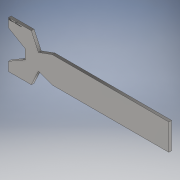
# Autodesk Inventor part: Spare Blade (In Blade Holder)
Saved by Autodesk Inventor 2021 (Build 250183000, 183)
## iProperties
Created: 2021-05-04
Part Number: Spare Blade (In Blade Holder)
Material: Generic
Document SubType Name: Modeling
Designer: AHUJA
Density: 1 g/cm^3
Appearance: Default
Author: AHUJA
Autodesk Inventor part; units mm, degrees
ref_plane "YZ Plane" through (0, 0, 0) normal (1, 0, 0) x (0, 1, 0)
ref_plane "XZ Plane" through (0, 0, 0) normal (0, 1, 0) x (-1, 0, 0)
ref_plane "XY Plane" through (0, 0, 0) normal (0, 0, 1) x (1, 0, 0)
sketch "Sketch1" plane through (0, 0, 0) normal (0, 0, 1) x (1, 0, 0)
  line L0 (0, 0) -> (80, 0)
  line L1 (80, 0) -> (80, 18)
  line L2 (80, 18) -> (0, 18)
  line L3 (0, 18) -> (0, 0)
  line L4 (0, 25) -> (-30, 25)
  line L5 (-30, -7) -> (0, -7)
  line L6 (0, -7) -> (0, 25)
  line L7 (0, 18) -> (-9.3969, 14.5798)
  line L8 (0, 18) -> (10, 18) construction
  line L9 (0, 0) -> (-9.3969, 3.4202)
  line L10 (0, 0) -> (10, 0) construction
  line L11 (-9.3969, 14.5798) -> (-14.2559, 25)
  line L12 (-9.3969, 14.5798) -> (2.1005, 14.5798) construction
  line L13 (-9.3969, 3.4202) -> (-14.2559, -7)
  line L14 (-9.3969, 3.4202) -> (2.1005, 3.4202) construction
  line L15 (-30, 25) -> (-30, 19)
  line L16 (-30, 19) -> (-18.3849, 12.294)
  line L17 (-30, -7) -> (-30, -1)
  line L18 (-30, -1) -> (-18.3849, 5.706)
  line L19 (-18.3849, 5.706) -> (-18.3849, 12.294)
  line L20 (-30, 25) -> (-30, 19)
  line L21 (-30, -1) -> (-30, -7)
  dimension "d0" = 80
  dimension "d1" = 18
  dimension "d2" = 30
  dimension "d3" = 0
  dimension "d4" = 7
  dimension "d5" = 7
  dimension "d6" = 160
  dimension "d7" = 160
  dimension "d8" = 10
  dimension "d9" = 10
  dimension "d10" = 115
  dimension "d11" = 115
  dimension "d12" = 6
  dimension "d13" = 120
  dimension "d14" = 6
  dimension "d15" = 120
  dimension "d16" = 30
  constraints: 44 end point, 6 horizontal, 6 parallel, 4 equal length, 3 perpendicular, 2 point on line
  measures "d0" distance of L1.end L2.end
  measures "d1" distance of L0.end L1.end
  measures "d2" distance of L4.start L4.end
  measures "d3" distance between parallel lines of L3 L6
  measures "d4" distance between parallel lines of L2 L4
  measures "d5" distance between parallel lines of L5 L0
  measures "d6" angle of L7 L8
  measures "d7" angle of L10 L9
  measures "d8" distance of L2.end L7.end
  measures "d9" distance of L0.start L9.end
  measures "d10" angle of L12 L11
  measures "d11" angle of L13 L14
  measures "d12" distance of L4.end L15.end
  measures "d13" angle of L16 L15
  measures "d14" distance of L5.start L17.end
  measures "d15" angle of L17 L18
  measures "d16" distance of L5.start L5.end
extrude "Extrusion1" add sketch "Sketch1" along normal blind 1.905 contours L3 L2 L1 L0 | L9 L13 L5 L17 L18 L19 L16 L15 L4 L11 L7 L3
sketch "Sketch2" plane through (0, 0, 1.905) normal (0, 0, 1) x (1, 0, 0)
  line L0 (-30.0598, 24.874) -> (-18.1328, 24.874) construction
  line L1 (-18.1328, 24.874) -> (-18.1328, 20.2492) construction
  line L2 (-18.1328, 20.2492) -> (-30.0598, 20.2492) construction
  line L3 (-30.0598, 20.2492) -> (-30.0598, 24.874) construction
  spline S0 degree 2 poles (-29.0996, 24.3152) (-28.6048, 24.816) (-28.4664, 24.816) knots 0 0 0 1 1 1
  spline S1 degree 2 poles (-28.4664, 24.816) (-28.4084, 24.816) (-28.4084, 24.7615) knots 0 0 0 1 1 1
  spline S2 degree 2 poles (-28.4084, 24.7615) (-28.4084, 24.7105) (-28.4499, 24.6482) knots 0 0 0 1 1 1
  spline S3 degree 2 poles (-28.4499, 24.6482) (-28.4811, 24.6041) (-28.8236, 24.2451) knots 0 0 0 1 1 1
  spline S4 degree 2 poles (-28.8236, 24.2451) (-29.1091, 23.9285) (-29.1091, 23.8731) knots 0 0 0 1 1 1
  spline S5 degree 2 poles (-29.1091, 23.8731) (-29.1091, 23.8541) (-29.0538, 23.8498) (-29.0538, 23.8437) knots 0 0 0 1 2 2 2
  spline S6 degree 2 poles (-29.0538, 23.8437) (-29.0538, 23.8238) (-29.097, 23.8238) knots 0 0 0 1 1 1
  spline S7 degree 2 poles (-29.097, 23.8238) (-29.1584, 23.8238) (-29.1584, 23.8818) knots 0 0 0 1 1 1
  spline S8 degree 2 poles (-29.1584, 23.8818) (-29.1584, 23.989) (-28.892, 24.2857) knots 0 0 0 1 1 1
  spline S9 degree 2 poles (-28.892, 24.2857) (-28.7986, 24.3904) (-28.5382, 24.6517) knots 0 0 0 1 1 1
  spline S10 degree 2 poles (-28.5382, 24.6517) (-28.4491, 24.7399) (-28.4491, 24.7754) knots 0 0 0 1 1 1
  spline S11 degree 2 poles (-28.4491, 24.7754) (-28.4491, 24.7892) (-28.4629, 24.7892) knots 0 0 0 1 1 1
  spline S12 degree 2 poles (-28.4629, 24.7892) (-28.5122, 24.7892) (-28.7406, 24.5998) knots 0 0 0 1 1 1
  spline S13 degree 2 poles (-28.7406, 24.5998) (-28.9231, 24.4475) (-29.0131, 24.3575) knots 0 0 0 1 1 1
  spline S14 degree 2 poles (-29.0131, 24.3575) (-29.0996, 24.271) (-29.2406, 24.1136) knots 0 0 0 1 1 1
  spline S15 degree 2 poles (-29.2406, 24.1136) (-29.4941, 23.829) (-29.5018, 23.829) knots 0 0 0 1 1 1
  spline S16 degree 2 poles (-29.5018, 23.829) (-29.5122, 23.829) (-29.5416, 23.8558) (-29.5416, 23.8671) knots 0 0 0 1 2 2 2
  spline S17 degree 2 poles (-29.5416, 23.8671) (-29.5416, 23.8947) (-28.9352, 24.611) (-28.9352, 24.6681) knots 0 0 0 1 2 2 2
  spline S18 degree 2 poles (-28.9352, 24.6681) (-28.9352, 24.6828) (-28.9491, 24.6828) knots 0 0 0 1 1 1
  spline S19 degree 2 poles (-28.9491, 24.6828) (-28.9863, 24.6828) (-29.1377, 24.5686) knots 0 0 0 1 1 1
  spline S20 degree 2 poles (-29.1377, 24.5686) (-29.2778, 24.4631) (-29.4456, 24.303) knots 0 0 0 1 1 1
  line L4 (-29.4456, 24.303) -> (-29.7345, 24.0167)
  line L5 (-29.7345, 24.0167) -> (-29.8358, 23.9077)
  spline S21 degree 2 poles (-29.8358, 23.9077) (-29.9205, 23.816) (-29.9275, 23.816) knots 0 0 0 1 1 1
  spline S22 degree 2 poles (-29.9275, 23.816) (-29.9387, 23.816) (-29.956, 23.8273) knots 0 0 0 1 1 1
  spline S23 degree 2 poles (-29.956, 23.8273) (-29.975, 23.8394) (-29.975, 23.8506) knots 0 0 0 1 1 1
  spline S24 degree 2 poles (-29.975, 23.8506) (-29.975, 23.874) (-29.796, 24.0747) knots 0 0 0 1 1 1
  line L6 (-29.796, 24.0747) -> (-29.4621, 24.4501)
  spline S25 degree 2 poles (-29.4621, 24.4501) (-29.2821, 24.6612) (-29.2821, 24.7113) knots 0 0 0 1 1 1
  spline S26 degree 2 poles (-29.2821, 24.7113) (-29.2821, 24.7295) (-29.3003, 24.7295) knots 0 0 0 1 1 1
  spline S27 degree 2 poles (-29.3003, 24.7295) (-29.3522, 24.7295) (-29.5148, 24.5972) knots 0 0 0 1 1 1
  spline S28 degree 2 poles (-29.5148, 24.5972) (-29.6368, 24.4985) (-29.8626, 24.2477) knots 0 0 0 1 1 1
  spline S29 degree 2 poles (-29.8626, 24.2477) (-29.8773, 24.2321) (-29.8859, 24.2321) knots 0 0 0 1 1 1
  spline S30 degree 2 poles (-29.8859, 24.2321) (-29.9015, 24.2321) (-29.9015, 24.2442) knots 0 0 0 1 1 1
  spline S31 degree 2 poles (-29.9015, 24.2442) (-29.9015, 24.2624) (-29.7769, 24.406) knots 0 0 0 1 1 1
  spline S32 degree 2 poles (-29.7769, 24.406) (-29.687, 24.5072) (-29.5512, 24.6205) knots 0 0 0 1 1 1
  spline S33 degree 2 poles (-29.5512, 24.6205) (-29.3747, 24.7658) (-29.296, 24.7658) knots 0 0 0 1 1 1
  spline S34 degree 2 poles (-29.296, 24.7658) (-29.2432, 24.7658) (-29.2432, 24.7079) knots 0 0 0 1 1 1
  spline S35 degree 2 poles (-29.2432, 24.7079) (-29.2432, 24.611) (-29.5001, 24.297) knots 0 0 0 1 1 1
  spline S36 degree 2 poles (-29.5001, 24.297) (-29.0615, 24.7148) (-28.9491, 24.7148) knots 0 0 0 1 1 1
  spline S37 degree 2 poles (-28.9491, 24.7148) (-28.8963, 24.7148) (-28.8963, 24.6603) knots 0 0 0 1 1 1
  spline S38 degree 2 poles (-28.8963, 24.6603) (-28.8963, 24.5747) (-29.0996, 24.3152) knots 0 0 0 1 1 1
  spline S39 degree 2 poles (-28.6091, 23.8722) (-28.6091, 23.8532) (-28.5676, 23.8532) knots 0 0 0 1 1 1
  spline S40 degree 2 poles (-28.5676, 23.8532) (-28.5581, 23.8532) (-28.5581, 23.8411) knots 0 0 0 1 1 1
  spline S41 degree 2 poles (-28.5581, 23.8411) (-28.5581, 23.8273) (-28.6057, 23.8273) knots 0 0 0 1 1 1
  spline S42 degree 2 poles (-28.6057, 23.8273) (-28.6593, 23.8273) (-28.6593, 23.8783) knots 0 0 0 1 1 1
  spline S43 degree 2 poles (-28.6593, 23.8783) (-28.6593, 23.9389) (-28.5001, 24.1292) knots 0 0 0 1 1 1
  line L7 (-28.5001, 24.1292) -> (-28.6948, 23.97)
  spline S44 degree 2 poles (-28.6948, 23.97) (-28.8678, 23.829) (-28.9456, 23.829) knots 0 0 0 1 1 1
  spline S45 degree 2 poles (-28.9456, 23.829) (-28.9543, 23.829) (-28.9543, 23.8385) knots 0 0 0 1 1 1
  spline S46 degree 2 poles (-28.9543, 23.8385) (-28.9543, 23.8523) (-28.9396, 23.8549) knots 0 0 0 1 1 1
  spline S47 degree 2 poles (-28.9396, 23.8549) (-28.8954, 23.8636) (-28.8582, 23.8844) knots 0 0 0 1 1 1
  spline S48 degree 2 poles (-28.8582, 23.8844) (-28.8115, 23.9094) (-28.661, 24.0288) knots 0 0 0 1 1 1
  line L8 (-28.661, 24.0288) -> (-28.443, 24.2113)
  spline S49 degree 2 poles (-28.443, 24.2113) (-28.4283, 24.2165) (-28.4041, 24.2165) knots 0 0 0 1 1 1
  spline S50 degree 2 poles (-28.4041, 24.2165) (-28.3799, 24.2165) (-28.3799, 24.1889) knots 0 0 0 1 1 1
  spline S51 degree 2 poles (-28.3799, 24.1889) (-28.3799, 24.1586) (-28.6091, 23.8956) (-28.6091, 23.8722) knots 0 0 0 1 2 2 2
  spline S52 degree 2 poles (-28.2942, 24.3662) (-28.3288, 24.3662) (-28.3288, 24.4008) knots 0 0 0 1 1 1
  spline S53 degree 2 poles (-28.3288, 24.4008) (-28.3288, 24.4302) (-28.2942, 24.4536) knots 0 0 0 1 1 1
  spline S54 degree 2 poles (-28.2942, 24.4536) (-28.2622, 24.4752) (-28.2311, 24.4752) knots 0 0 0 1 1 1
  spline S55 degree 2 poles (-28.2311, 24.4752) (-28.1939, 24.4752) (-28.1939, 24.4345) knots 0 0 0 1 1 1
  spline S56 degree 2 poles (-28.1939, 24.4345) (-28.1939, 24.4051) (-28.2311, 24.3844) knots 0 0 0 1 1 1
  spline S57 degree 2 poles (-28.2311, 24.3844) (-28.2631, 24.3662) (-28.2942, 24.3662) knots 0 0 0 1 1 1
  line L9 (-28.0935, 24.1586) -> (-28.2847, 23.9977)
  line L10 (-28.2847, 23.9977) -> (-28.4162, 23.8947)
  spline S58 degree 2 poles (-28.4162, 23.8947) (-28.5096, 23.829) (-28.5693, 23.829) knots 0 0 0 1 1 1
  spline S59 degree 2 poles (-28.5693, 23.829) (-28.578, 23.829) (-28.578, 23.8385) knots 0 0 0 1 1 1
  spline S60 degree 2 poles (-28.578, 23.8385) (-28.578, 23.8515) (-28.5633, 23.8549) knots 0 0 0 1 1 1
  spline S61 degree 2 poles (-28.5633, 23.8549) (-28.4698, 23.8774) (-28.3089, 24.0107) knots 0 0 0 1 1 1
  line L11 (-28.3089, 24.0107) -> (-28.1057, 24.1802)
  spline S62 degree 2 poles (-28.1057, 24.1802) (-28.0356, 24.239) (-27.8799, 24.412) knots 0 0 0 1 1 1
  line L12 (-27.8799, 24.412) -> (-27.68, 24.6404)
  spline S63 degree 2 poles (-27.68, 24.6404) (-27.6325, 24.6966) (-27.6134, 24.6966) knots 0 0 0 1 1 1
  spline S64 degree 2 poles (-27.6134, 24.6966) (-27.5884, 24.6966) (-27.5884, 24.6716) knots 0 0 0 1 1 1
  spline S65 degree 2 poles (-27.5884, 24.6716) (-27.5884, 24.6404) (-27.6498, 24.5643) knots 0 0 0 1 1 1
  line L13 (-27.6498, 24.5643) -> (-27.738, 24.4639)
  line L14 (-27.738, 24.4639) -> (-28.0226, 24.1361)
  spline S66 degree 2 poles (-28.0226, 24.1361) (-27.9179, 24.2113) (-27.8686, 24.2113) knots 0 0 0 1 1 1
  spline S67 degree 2 poles (-27.8686, 24.2113) (-27.8107, 24.2113) (-27.8107, 24.1543) knots 0 0 0 1 1 1
  spline S68 degree 2 poles (-27.8107, 24.1543) (-27.8107, 24.0902) (-27.9231, 24.0444) knots 0 0 0 1 1 1
  spline S69 degree 2 poles (-27.9231, 24.0444) (-28.0148, 24.0072) (-28.0935, 24.0063) knots 0 0 0 1 1 1
  spline S70 degree 2 poles (-28.0935, 24.0063) (-28.0685, 23.9458) (-28.0278, 23.8688) knots 0 0 0 1 1 1
  spline S71 degree 2 poles (-28.0278, 23.8688) (-28.014, 23.8523) (-27.9837, 23.8523) knots 0 0 0 1 1 1
  spline S72 degree 2 poles (-27.9837, 23.8523) (-27.9733, 23.8523) (-27.9733, 23.8411) knots 0 0 0 1 1 1
  spline S73 degree 2 poles (-27.9733, 23.8411) (-27.9733, 23.8255) (-28.0287, 23.8255) knots 0 0 0 1 1 1
  spline S74 degree 2 poles (-28.0287, 23.8255) (-28.0563, 23.8255) (-28.0754, 23.8394) knots 0 0 0 1 1 1
  spline S75 degree 2 poles (-28.0754, 23.8394) (-28.0927, 23.8515) (-28.1532, 23.9804) knots 0 0 0 1 1 1
  line L15 (-28.1532, 23.9804) -> (-28.225, 23.8947)
  spline S76 degree 2 poles (-28.225, 23.8947) (-28.2847, 23.8247) (-28.2968, 23.8247) knots 0 0 0 1 1 1
  spline S77 degree 2 poles (-28.2968, 23.8247) (-28.3271, 23.8247) (-28.3271, 23.8601) knots 0 0 0 1 1 1
  spline S78 degree 2 poles (-28.3271, 23.8601) (-28.3271, 23.8809) (-28.2146, 24.0167) knots 0 0 0 1 1 1
  line L16 (-28.2146, 24.0167) -> (-28.0935, 24.1586)
  spline S79 degree 2 poles (-28.1152, 24.0228) (-28.0088, 24.0366) (-27.8704, 24.1266) (-27.8704, 24.1586) knots 0 0 0 1 2 2 2
  spline S80 degree 2 poles (-27.8704, 24.1586) (-27.8704, 24.175) (-27.8911, 24.175) knots 0 0 0 1 1 1
  spline S81 degree 2 poles (-27.8911, 24.175) (-27.969, 24.175) (-28.1152, 24.0228) knots 0 0 0 1 1 1
  spline S82 degree 2 poles (-27.7216, 23.9795) (-27.9127, 23.829) (-27.9845, 23.829) knots 0 0 0 1 1 1
  spline S83 degree 2 poles (-27.9845, 23.829) (-27.9932, 23.829) (-27.9932, 23.8385) knots 0 0 0 1 1 1
  spline S84 degree 2 poles (-27.9932, 23.8385) (-27.9932, 23.8523) (-27.9759, 23.8549) knots 0 0 0 1 1 1
  spline S85 degree 2 poles (-27.9759, 23.8549) (-27.9093, 23.8653) (-27.7899, 23.9587) knots 0 0 0 1 1 1
  line L17 (-27.7899, 23.9587) -> (-27.6982, 24.0305)
  line L18 (-27.6982, 24.0305) -> (-27.5503, 24.1482)
  spline S86 degree 2 poles (-27.5503, 24.1482) (-27.4491, 24.2183) (-27.3764, 24.2183) knots 0 0 0 1 1 1
  spline S87 degree 2 poles (-27.3764, 24.2183) (-27.3228, 24.2183) (-27.3167, 24.1646) knots 0 0 0 1 1 1
  spline S88 degree 2 poles (-27.3167, 24.1646) (-27.289, 24.1914) (-27.2778, 24.1914) knots 0 0 0 1 1 1
  spline S89 degree 2 poles (-27.2778, 24.1914) (-27.2544, 24.1914) (-27.2544, 24.1716) knots 0 0 0 1 1 1
  spline S90 degree 2 poles (-27.2544, 24.1716) (-27.2544, 24.1465) (-27.4733, 23.8913) (-27.4733, 23.8696) knots 0 0 0 1 2 2 2
  spline S91 degree 2 poles (-27.4733, 23.8696) (-27.4733, 23.8549) (-27.4275, 23.8532) (-27.4275, 23.842) knots 0 0 0 1 2 2 2
  spline S92 degree 2 poles (-27.4275, 23.842) (-27.4275, 23.8273) (-27.475, 23.8273) knots 0 0 0 1 1 1
  spline S93 degree 2 poles (-27.475, 23.8273) (-27.5226, 23.8273) (-27.5226, 23.8696) knots 0 0 0 1 1 1
  spline S94 degree 2 poles (-27.5226, 23.8696) (-27.5226, 23.9034) (-27.4845, 23.9648) knots 0 0 0 1 1 1
  line L19 (-27.4845, 23.9648) -> (-27.5728, 23.8895)
  spline S95 degree 2 poles (-27.5728, 23.8895) (-27.6377, 23.8411) (-27.6766, 23.8411) knots 0 0 0 1 1 1
  spline S96 degree 2 poles (-27.6766, 23.8411) (-27.738, 23.8411) (-27.738, 23.9034) knots 0 0 0 1 1 1
  spline S97 degree 2 poles (-27.738, 23.9034) (-27.738, 23.938) (-27.7216, 23.9795) knots 0 0 0 1 1 1
  spline S98 degree 2 poles (-27.3669, 24.1889) (-27.4093, 24.1889) (-27.6731, 23.9371) (-27.6731, 23.8947) knots 0 0 0 1 2 2 2
  spline S99 degree 2 poles (-27.6731, 23.8947) (-27.6731, 23.8757) (-27.655, 23.8757) knots 0 0 0 1 1 1
  spline S100 degree 2 poles (-27.655, 23.8757) (-27.6134, 23.8757) (-27.3461, 24.1222) (-27.3461, 24.1655) knots 0 0 0 1 2 2 2
  spline S101 degree 2 poles (-27.3461, 24.1655) (-27.3461, 24.1889) (-27.3669, 24.1889) knots 0 0 0 1 1 1
  spline S102 degree 2 poles (-27.2129, 23.951) (-27.3617, 23.829) (-27.4387, 23.829) knots 0 0 0 1 1 1
  spline S103 degree 2 poles (-27.4387, 23.829) (-27.4473, 23.829) (-27.4473, 23.8376) knots 0 0 0 1 1 1
  spline S104 degree 2 poles (-27.4473, 23.8376) (-27.4473, 23.8515) (-27.4326, 23.8549) knots 0 0 0 1 1 1
  spline S105 degree 2 poles (-27.4326, 23.8549) (-27.4067, 23.861) (-27.3513, 23.8835) knots 0 0 0 1 1 1
  spline S106 degree 2 poles (-27.3513, 23.8835) (-27.3003, 23.9112) (-27.0901, 24.0859) knots 0 0 0 1 1 1
  spline S107 degree 2 poles (-27.0901, 24.0859) (-26.8911, 24.2511) (-26.8859, 24.2511) knots 0 0 0 1 1 1
  spline S108 degree 2 poles (-26.8859, 24.2511) (-26.8695, 24.2511) (-26.8375, 24.2226) (-26.8375, 24.2062) knots 0 0 0 1 2 2 2
  spline S109 degree 2 poles (-26.8375, 24.2062) (-26.8375, 24.1543) (-26.9188, 24.0228) knots 0 0 0 1 1 1
  spline S110 degree 2 poles (-26.9188, 24.0228) (-26.9897, 23.9094) (-27.0425, 23.8532) knots 0 0 0 1 1 1
  spline S111 degree 2 poles (-27.0425, 23.8532) (-27.0114, 23.8532) (-27.0114, 23.842) knots 0 0 0 1 1 1
  spline S112 degree 2 poles (-27.0114, 23.842) (-27.0114, 23.8273) (-27.0416, 23.8273) knots 0 0 0 1 1 1
  spline S113 degree 2 poles (-27.0416, 23.8273) (-27.0494, 23.8273) (-27.0797, 23.8325) (-27.0884, 23.8325) knots 0 0 0 1 2 2 2
  spline S114 degree 2 poles (-27.0884, 23.8325) (-27.0935, 23.8325) (-27.1169, 23.8281) (-27.1221, 23.8281) knots 0 0 0 1 2 2 2
  spline S115 degree 2 poles (-27.1221, 23.8281) (-27.2129, 23.8281) (-27.2129, 23.951) knots 0 0 0 1 1 1
  spline S116 degree 2 poles (-27.0996, 23.8878) (-27.0494, 23.9293) (-26.9897, 24.0314) knots 0 0 0 1 1 1
  spline S117 degree 2 poles (-26.9897, 24.0314) (-26.9344, 24.1257) (-26.9119, 24.1984) knots 0 0 0 1 1 1
  line L20 (-26.9119, 24.1984) -> (-27.1671, 23.9908)
  spline S118 degree 2 poles (-27.1671, 23.9908) (-27.1411, 23.9864) (-27.123, 23.9492) knots 0 0 0 1 1 1
  line L21 (-27.123, 23.9492) -> (-27.0996, 23.8878)
  line L22 (-27.1195, 23.8662) -> (-27.1394, 23.9233)
  spline S119 degree 2 poles (-27.1394, 23.9233) (-27.1558, 23.9648) (-27.1705, 23.9648) knots 0 0 0 1 1 1
  spline S120 degree 2 poles (-27.1705, 23.9648) (-27.1861, 23.9648) (-27.1861, 23.9406) knots 0 0 0 1 1 1
  spline S121 degree 2 poles (-27.1861, 23.9406) (-27.1861, 23.9155) (-27.1723, 23.8895) knots 0 0 0 1 1 1
  spline S122 degree 2 poles (-27.1723, 23.8895) (-27.1558, 23.8601) (-27.1333, 23.8601) knots 0 0 0 1 1 1
  spline S123 degree 2 poles (-27.1333, 23.8601) (-27.1247, 23.8601) (-27.1195, 23.8662) knots 0 0 0 1 1 1
  spline S124 degree 2 poles (-26.7596, 23.9795) (-26.9508, 23.829) (-27.0226, 23.829) knots 0 0 0 1 1 1
  spline S125 degree 2 poles (-27.0226, 23.829) (-27.0313, 23.829) (-27.0313, 23.8385) knots 0 0 0 1 1 1
  spline S126 degree 2 poles (-27.0313, 23.8385) (-27.0313, 23.8523) (-27.014, 23.8549) knots 0 0 0 1 1 1
  spline S127 degree 2 poles (-27.014, 23.8549) (-26.9473, 23.8653) (-26.828, 23.9587) knots 0 0 0 1 1 1
  line L23 (-26.828, 23.9587) -> (-26.7363, 24.0305)
  line L24 (-26.7363, 24.0305) -> (-26.5884, 24.1482)
  spline S128 degree 2 poles (-26.5884, 24.1482) (-26.4871, 24.2183) (-26.4145, 24.2183) knots 0 0 0 1 1 1
  spline S129 degree 2 poles (-26.4145, 24.2183) (-26.3608, 24.2183) (-26.3548, 24.1646) knots 0 0 0 1 1 1
  spline S130 degree 2 poles (-26.3548, 24.1646) (-26.3271, 24.1914) (-26.3159, 24.1914) knots 0 0 0 1 1 1
  spline S131 degree 2 poles (-26.3159, 24.1914) (-26.2925, 24.1914) (-26.2925, 24.1716) knots 0 0 0 1 1 1
  spline S132 degree 2 poles (-26.2925, 24.1716) (-26.2925, 24.1465) (-26.5114, 23.8913) (-26.5114, 23.8696) knots 0 0 0 1 2 2 2
  spline S133 degree 2 poles (-26.5114, 23.8696) (-26.5114, 23.8549) (-26.4655, 23.8532) (-26.4655, 23.842) knots 0 0 0 1 2 2 2
  spline S134 degree 2 poles (-26.4655, 23.842) (-26.4655, 23.8273) (-26.5131, 23.8273) knots 0 0 0 1 1 1
  spline S135 degree 2 poles (-26.5131, 23.8273) (-26.5607, 23.8273) (-26.5607, 23.8696) knots 0 0 0 1 1 1
  spline S136 degree 2 poles (-26.5607, 23.8696) (-26.5607, 23.9034) (-26.5226, 23.9648) knots 0 0 0 1 1 1
  line L25 (-26.5226, 23.9648) -> (-26.6108, 23.8895)
  spline S137 degree 2 poles (-26.6108, 23.8895) (-26.6757, 23.8411) (-26.7146, 23.8411) knots 0 0 0 1 1 1
  spline S138 degree 2 poles (-26.7146, 23.8411) (-26.7761, 23.8411) (-26.7761, 23.9034) knots 0 0 0 1 1 1
  spline S139 degree 2 poles (-26.7761, 23.9034) (-26.7761, 23.938) (-26.7596, 23.9795) knots 0 0 0 1 1 1
  spline S140 degree 2 poles (-26.405, 24.1889) (-26.4473, 24.1889) (-26.7112, 23.9371) (-26.7112, 23.8947) knots 0 0 0 1 2 2 2
  spline S141 degree 2 poles (-26.7112, 23.8947) (-26.7112, 23.8757) (-26.693, 23.8757) knots 0 0 0 1 1 1
  spline S142 degree 2 poles (-26.693, 23.8757) (-26.6515, 23.8757) (-26.3842, 24.1222) (-26.3842, 24.1655) knots 0 0 0 1 2 2 2
  spline S143 degree 2 poles (-26.3842, 24.1655) (-26.3842, 24.1889) (-26.405, 24.1889) knots 0 0 0 1 1 1
  line L26 (-24.8721, 24.2408) -> (-24.8072, 24.2408)
  spline S144 degree 2 poles (-24.8072, 24.2408) (-24.7596, 24.2356) (-24.7596, 24.2113) knots 0 0 0 1 1 1
  spline S145 degree 2 poles (-24.7596, 24.2113) (-24.7596, 24.1958) (-24.7942, 24.1958) knots 0 0 0 1 1 1
  line L27 (-24.7942, 24.1958) -> (-24.8401, 24.1984)
  line L28 (-24.8401, 24.1984) -> (-24.9076, 24.1975)
  line L29 (-24.9076, 24.1975) -> (-25.0529, 24.0132)
  spline S146 degree 2 poles (-25.0529, 24.0132) (-25.2008, 23.829) (-25.2164, 23.829) knots 0 0 0 1 1 1
  spline S147 degree 2 poles (-25.2164, 23.829) (-25.2302, 23.829) (-25.2415, 23.8498) knots 0 0 0 1 1 1
  spline S148 degree 2 poles (-25.2415, 23.8498) (-25.2527, 23.8671) (-25.2527, 23.8818) knots 0 0 0 1 1 1
  spline S149 degree 2 poles (-25.2527, 23.8818) (-25.2527, 23.9043) (-25.0096, 24.1975) knots 0 0 0 1 1 1
  line L30 (-25.0096, 24.1975) -> (-25.065, 24.1975)
  spline S150 degree 2 poles (-25.065, 24.1975) (-25.1818, 24.1966) (-25.4119, 24.1854) knots 0 0 0 1 1 1
  line L31 (-25.4119, 24.1854) -> (-25.6524, 23.9786)
  line L32 (-25.6524, 23.9786) -> (-25.7467, 23.8947)
  spline S151 degree 2 poles (-25.7467, 23.8947) (-25.8219, 23.829) (-25.8384, 23.829) knots 0 0 0 1 1 1
  spline S152 degree 2 poles (-25.8384, 23.829) (-25.8582, 23.829) (-25.8582, 23.8498) knots 0 0 0 1 1 1
  spline S153 degree 2 poles (-25.8582, 23.8498) (-25.8582, 23.8757) (-25.6524, 24.0478) knots 0 0 0 1 1 1
  line L33 (-25.6524, 24.0478) -> (-25.4889, 24.1837)
  spline S154 degree 2 poles (-25.4889, 24.1837) (-25.8159, 24.1681) (-25.8262, 24.1499) knots 0 0 0 1 1 1
  line L34 (-25.8262, 24.1499) -> (-25.8262, 24.1491)
  spline S155 degree 2 poles (-25.8262, 24.1491) (-25.8262, 24.1352) (-25.7242, 24.1352) knots 0 0 0 1 1 1
  line L35 (-25.7242, 24.1352) -> (-25.629, 24.1369)
  spline S156 degree 2 poles (-25.629, 24.1369) (-25.61, 24.1369) (-25.61, 24.1283) knots 0 0 0 1 1 1
  spline S157 degree 2 poles (-25.61, 24.1283) (-25.61, 24.1084) (-25.7657, 24.1084) knots 0 0 0 1 1 1
  spline S158 degree 2 poles (-25.7657, 24.1084) (-25.898, 24.1084) (-25.898, 24.1421) knots 0 0 0 1 1 1
  spline S159 degree 2 poles (-25.898, 24.1421) (-25.898, 24.1854) (-25.8193, 24.2018) knots 0 0 0 1 1 1
  spline S160 degree 2 poles (-25.8193, 24.2018) (-25.7977, 24.2062) (-25.7095, 24.2122) knots 0 0 0 1 1 1
  line L36 (-25.7095, 24.2122) -> (-25.4318, 24.2304)
  spline S161 degree 2 poles (-25.4318, 24.2304) (-25.2631, 24.3696) (-24.9499, 24.592) knots 0 0 0 1 1 1
  spline S162 degree 2 poles (-24.9499, 24.592) (-24.5512, 24.874) (-24.4742, 24.874) knots 0 0 0 1 1 1
  spline S163 degree 2 poles (-24.4742, 24.874) (-24.4352, 24.874) (-24.4352, 24.8238) knots 0 0 0 1 1 1
  spline S164 degree 2 poles (-24.4352, 24.8238) (-24.4352, 24.7814) (-24.5356, 24.6568) knots 0 0 0 1 1 1
  line L37 (-24.5356, 24.6568) -> (-24.8721, 24.2408)
  line L38 (-24.9742, 24.2408) -> (-24.6403, 24.6465)
  line L39 (-24.6403, 24.6465) -> (-24.578, 24.7226)
  spline S165 degree 2 poles (-24.578, 24.7226) (-24.5382, 24.7728) (-24.5252, 24.8004) knots 0 0 0 1 1 1
  line L40 (-24.5252, 24.8004) -> (-24.5243, 24.803)
  spline S166 degree 2 poles (-24.5243, 24.803) (-24.5243, 24.8108) (-24.5313, 24.8108) knots 0 0 0 1 1 1
  spline S167 degree 2 poles (-24.5313, 24.8108) (-24.565, 24.8108) (-24.956, 24.5254) knots 0 0 0 1 1 1
  line L41 (-24.956, 24.5254) -> (-25.3479, 24.2338)
  line L42 (-25.3479, 24.2338) -> (-24.9742, 24.2408)
  line L43 (-24.6775, 24.028) -> (-24.8262, 23.9112)
  spline S168 degree 2 poles (-24.8262, 23.9112) (-24.9422, 23.829) (-25.0027, 23.829) knots 0 0 0 1 1 1
  spline S169 degree 2 poles (-25.0027, 23.829) (-25.0114, 23.829) (-25.0114, 23.8376) knots 0 0 0 1 1 1
  spline S170 degree 2 poles (-25.0114, 23.8376) (-25.0114, 23.8515) (-24.9941, 23.8549) knots 0 0 0 1 1 1
  spline S171 degree 2 poles (-24.9941, 23.8549) (-24.9275, 23.8679) (-24.8141, 23.9536) knots 0 0 0 1 1 1
  line L44 (-24.8141, 23.9536) -> (-24.616, 24.1119)
  spline S172 degree 2 poles (-24.616, 24.1119) (-24.4534, 24.2451) (-24.366, 24.2451) knots 0 0 0 1 1 1
  spline S173 degree 2 poles (-24.366, 24.2451) (-24.3193, 24.2451) (-24.3193, 24.2096) knots 0 0 0 1 1 1
  spline S174 degree 2 poles (-24.3193, 24.2096) (-24.3038, 24.2096) (-24.3038, 24.1958) knots 0 0 0 1 1 1
  spline S175 degree 2 poles (-24.3038, 24.1958) (-24.3038, 24.1837) (-24.3211, 24.1828) knots 0 0 0 1 1 1
  spline S176 degree 2 poles (-24.3211, 24.1828) (-24.3358, 24.1318) (-24.3747, 24.0816) knots 0 0 0 1 1 1
  spline S177 degree 2 poles (-24.3747, 24.0816) (-24.4223, 24.0219) (-24.4655, 24.0219) knots 0 0 0 1 1 1
  spline S178 degree 2 poles (-24.4655, 24.0219) (-24.4915, 24.0219) (-24.4915, 24.0453) knots 0 0 0 1 1 1
  spline S179 degree 2 poles (-24.4915, 24.0453) (-24.4915, 24.079) (-24.4361, 24.1326) knots 0 0 0 1 1 1
  spline S180 degree 2 poles (-24.4361, 24.1326) (-24.3868, 24.1802) (-24.3479, 24.1966) knots 0 0 0 1 1 1
  line L45 (-24.3479, 24.1966) -> (-24.3461, 24.2044)
  spline S181 degree 2 poles (-24.3461, 24.2044) (-24.3461, 24.2148) (-24.3565, 24.2148) knots 0 0 0 1 1 1
  spline S182 degree 2 poles (-24.3565, 24.2148) (-24.4024, 24.2148) (-24.6506, 23.9596) (-24.6506, 23.9086) knots 0 0 0 1 2 2 2
  spline S183 degree 2 poles (-24.6506, 23.9086) (-24.6506, 23.8766) (-24.623, 23.8645) knots 0 0 0 1 1 1
  spline S184 degree 2 poles (-24.623, 23.8645) (-24.6091, 23.8575) (-24.5719, 23.8541) knots 0 0 0 1 1 1
  spline S185 degree 2 poles (-24.5719, 23.8541) (-24.5442, 23.8515) (-24.5442, 23.842) knots 0 0 0 1 1 1
  spline S186 degree 2 poles (-24.5442, 23.842) (-24.5442, 23.8273) (-24.5944, 23.8273) knots 0 0 0 1 1 1
  spline S187 degree 2 poles (-24.5944, 23.8273) (-24.706, 23.8273) (-24.706, 23.9285) knots 0 0 0 1 1 1
  spline S188 degree 2 poles (-24.706, 23.9285) (-24.706, 23.9665) (-24.6775, 24.028) knots 0 0 0 1 1 1
  spline S189 degree 2 poles (-24.3591, 24.1646) (-24.3799, 24.1551) (-24.4179, 24.1179) knots 0 0 0 1 1 1
  spline S190 degree 2 poles (-24.4179, 24.1179) (-24.4586, 24.0781) (-24.4586, 24.0626) knots 0 0 0 1 1 1
  line L46 (-24.4586, 24.0626) -> (-24.4525, 24.0565)
  spline S191 degree 2 poles (-24.4525, 24.0565) (-24.4335, 24.0565) (-24.3989, 24.1006) knots 0 0 0 1 1 1
  spline S192 degree 2 poles (-24.3989, 24.1006) (-24.3704, 24.1387) (-24.3591, 24.1646) knots 0 0 0 1 1 1
  line L47 (-24.0797, 24.1586) -> (-24.2709, 23.9977)
  line L48 (-24.2709, 23.9977) -> (-24.4024, 23.8947)
  spline S193 degree 2 poles (-24.4024, 23.8947) (-24.4958, 23.829) (-24.5555, 23.829) knots 0 0 0 1 1 1
  spline S194 degree 2 poles (-24.5555, 23.829) (-24.5641, 23.829) (-24.5641, 23.8385) knots 0 0 0 1 1 1
  spline S195 degree 2 poles (-24.5641, 23.8385) (-24.5641, 23.8515) (-24.5494, 23.8549) knots 0 0 0 1 1 1
  spline S196 degree 2 poles (-24.5494, 23.8549) (-24.456, 23.8774) (-24.2951, 24.0107) knots 0 0 0 1 1 1
  line L49 (-24.2951, 24.0107) -> (-24.0918, 24.1802)
  spline S197 degree 2 poles (-24.0918, 24.1802) (-24.0217, 24.239) (-23.866, 24.412) knots 0 0 0 1 1 1
  line L50 (-23.866, 24.412) -> (-23.6662, 24.6404)
  spline S198 degree 2 poles (-23.6662, 24.6404) (-23.6186, 24.6966) (-23.5996, 24.6966) knots 0 0 0 1 1 1
  spline S199 degree 2 poles (-23.5996, 24.6966) (-23.5745, 24.6966) (-23.5745, 24.6716) knots 0 0 0 1 1 1
  spline S200 degree 2 poles (-23.5745, 24.6716) (-23.5745, 24.6404) (-23.6359, 24.5643) knots 0 0 0 1 1 1
  line L51 (-23.6359, 24.5643) -> (-23.7242, 24.4639)
  line L52 (-23.7242, 24.4639) -> (-24.0088, 24.1361)
  spline S201 degree 2 poles (-24.0088, 24.1361) (-23.9041, 24.2113) (-23.8548, 24.2113) knots 0 0 0 1 1 1
  spline S202 degree 2 poles (-23.8548, 24.2113) (-23.7968, 24.2113) (-23.7968, 24.1543) knots 0 0 0 1 1 1
  spline S203 degree 2 poles (-23.7968, 24.1543) (-23.7968, 24.0902) (-23.9093, 24.0444) knots 0 0 0 1 1 1
  spline S204 degree 2 poles (-23.9093, 24.0444) (-24.001, 24.0072) (-24.0797, 24.0063) knots 0 0 0 1 1 1
  spline S205 degree 2 poles (-24.0797, 24.0063) (-24.0546, 23.9458) (-24.014, 23.8688) knots 0 0 0 1 1 1
  spline S206 degree 2 poles (-24.014, 23.8688) (-24.0001, 23.8523) (-23.9698, 23.8523) knots 0 0 0 1 1 1
  spline S207 degree 2 poles (-23.9698, 23.8523) (-23.9595, 23.8523) (-23.9595, 23.8411) knots 0 0 0 1 1 1
  spline S208 degree 2 poles (-23.9595, 23.8411) (-23.9595, 23.8255) (-24.0148, 23.8255) knots 0 0 0 1 1 1
  spline S209 degree 2 poles (-24.0148, 23.8255) (-24.0425, 23.8255) (-24.0615, 23.8394) knots 0 0 0 1 1 1
  spline S210 degree 2 poles (-24.0615, 23.8394) (-24.0788, 23.8515) (-24.1394, 23.9804) knots 0 0 0 1 1 1
  line L53 (-24.1394, 23.9804) -> (-24.2112, 23.8947)
  spline S211 degree 2 poles (-24.2112, 23.8947) (-24.2709, 23.8247) (-24.283, 23.8247) knots 0 0 0 1 1 1
  spline S212 degree 2 poles (-24.283, 23.8247) (-24.3133, 23.8247) (-24.3133, 23.8601) knots 0 0 0 1 1 1
  spline S213 degree 2 poles (-24.3133, 23.8601) (-24.3133, 23.8809) (-24.2008, 24.0167) knots 0 0 0 1 1 1
  line L54 (-24.2008, 24.0167) -> (-24.0797, 24.1586)
  spline S214 degree 2 poles (-24.1013, 24.0228) (-23.9949, 24.0366) (-23.8565, 24.1266) (-23.8565, 24.1586) knots 0 0 0 1 2 2 2
  spline S215 degree 2 poles (-23.8565, 24.1586) (-23.8565, 24.175) (-23.8773, 24.175) knots 0 0 0 1 1 1
  spline S216 degree 2 poles (-23.8773, 24.175) (-23.9551, 24.175) (-24.1013, 24.0228) knots 0 0 0 1 1 1
  spline S217 degree 2 poles (-23.7043, 23.944) (-23.7397, 23.9354) (-23.8384, 23.8783) knots 0 0 0 1 1 1
  spline S218 degree 2 poles (-23.8384, 23.8783) (-23.9257, 23.829) (-23.9707, 23.829) knots 0 0 0 1 1 1
  spline S219 degree 2 poles (-23.9707, 23.829) (-23.9794, 23.829) (-23.9794, 23.8385) knots 0 0 0 1 1 1
  spline S220 degree 2 poles (-23.9794, 23.8385) (-23.9794, 23.8523) (-23.9612, 23.8549) knots 0 0 0 1 1 1
  spline S221 degree 2 poles (-23.9612, 23.8549) (-23.9171, 23.8619) (-23.8384, 23.9077) knots 0 0 0 1 1 1
  spline S222 degree 2 poles (-23.8384, 23.9077) (-23.751, 23.957) (-23.6956, 23.97) knots 0 0 0 1 1 1
  spline S223 degree 2 poles (-23.6956, 23.97) (-23.6627, 24.0496) (-23.5598, 24.1369) knots 0 0 0 1 1 1
  spline S224 degree 2 poles (-23.5598, 24.1369) (-23.4508, 24.2304) (-23.3738, 24.2304) knots 0 0 0 1 1 1
  spline S225 degree 2 poles (-23.3738, 24.2304) (-23.3167, 24.2304) (-23.3167, 24.1819) knots 0 0 0 1 1 1
  spline S226 degree 2 poles (-23.3167, 24.1819) (-23.3167, 24.1179) (-23.4378, 24.0427) knots 0 0 0 1 1 1
  spline S227 degree 2 poles (-23.4378, 24.0427) (-23.5261, 23.9873) (-23.6186, 23.9553) knots 0 0 0 1 1 1
  spline S228 degree 2 poles (-23.6186, 23.9553) (-23.629, 23.9328) (-23.629, 23.9086) knots 0 0 0 1 1 1
  spline S229 degree 2 poles (-23.629, 23.9086) (-23.629, 23.8714) (-23.6031, 23.8601) knots 0 0 0 1 1 1
  spline S230 degree 2 poles (-23.6031, 23.8601) (-23.5901, 23.8558) (-23.5546, 23.8541) knots 0 0 0 1 1 1
  spline S231 degree 2 poles (-23.5546, 23.8541) (-23.5287, 23.8532) (-23.5287, 23.8411) knots 0 0 0 1 1 1
  spline S232 degree 2 poles (-23.5287, 23.8411) (-23.5287, 23.8229) (-23.6169, 23.8229) knots 0 0 0 1 1 1
  spline S233 degree 2 poles (-23.6169, 23.8229) (-23.7095, 23.8229) (-23.7095, 23.9034) knots 0 0 0 1 1 1
  spline S234 degree 2 poles (-23.7095, 23.9034) (-23.7095, 23.9216) (-23.7043, 23.944) knots 0 0 0 1 1 1
  spline S235 degree 2 poles (-23.6108, 23.9847) (-23.5451, 24.0167) (-23.4716, 24.0721) knots 0 0 0 1 1 1
  spline S236 degree 2 poles (-23.4716, 24.0721) (-23.3747, 24.1439) (-23.3747, 24.1863) knots 0 0 0 1 1 1
  spline S237 degree 2 poles (-23.3747, 24.1863) (-23.3747, 24.2036) (-23.3903, 24.2036) knots 0 0 0 1 1 1
  spline S238 degree 2 poles (-23.3903, 24.2036) (-23.437, 24.2036) (-23.5166, 24.1179) knots 0 0 0 1 1 1
  spline S239 degree 2 poles (-23.5166, 24.1179) (-23.5884, 24.0392) (-23.6108, 23.9847) knots 0 0 0 1 1 1
  spline S240 degree 2 poles (-23.1377, 24.1447) (-23.1411, 24.1681) (-23.1411, 24.1733) knots 0 0 0 1 1 1
  spline S241 degree 2 poles (-23.1411, 24.1733) (-23.1411, 24.1923) (-23.0494, 24.2745) (-23.0321, 24.2745) knots 0 0 0 1 2 2 2
  spline S242 degree 2 poles (-23.0321, 24.2745) (-23.0157, 24.2745) (-23.0157, 24.2598) knots 0 0 0 1 1 1
  spline S243 degree 2 poles (-23.0157, 24.2598) (-23.0157, 24.2468) (-23.0339, 24.2165) knots 0 0 0 1 1 1
  spline S244 degree 2 poles (-23.0339, 24.2165) (-22.9525, 24.2165) (-22.9525, 24.1525) knots 0 0 0 1 1 1
  spline S245 degree 2 poles (-22.9525, 24.1525) (-22.9525, 24.1023) (-23.1602, 23.8809) (-23.1602, 23.8671) knots 0 0 0 1 2 2 2
  spline S246 degree 2 poles (-23.1602, 23.8671) (-23.1602, 23.8549) (-23.1463, 23.8532) knots 0 0 0 1 1 1
  line L55 (-23.1463, 23.8532) -> (-23.123, 23.8541)
  spline S247 degree 2 poles (-23.123, 23.8541) (-23.1134, 23.8541) (-23.1134, 23.842) knots 0 0 0 1 1 1
  spline S248 degree 2 poles (-23.1134, 23.842) (-23.1134, 23.8273) (-23.155, 23.8273) knots 0 0 0 1 1 1
  spline S249 degree 2 poles (-23.155, 23.8273) (-23.2077, 23.8273) (-23.2077, 23.874) knots 0 0 0 1 1 1
  spline S250 degree 2 poles (-23.2077, 23.874) (-23.2077, 23.9207) (-23.155, 23.9899) knots 0 0 0 1 1 1
  spline S251 degree 2 poles (-23.155, 23.9899) (-23.1221, 24.0331) (-23.0581, 24.098) knots 0 0 0 1 1 1
  spline S252 degree 2 poles (-23.0581, 24.098) (-23.0053, 24.1499) (-23.0053, 24.1551) knots 0 0 0 1 1 1
  spline S253 degree 2 poles (-23.0053, 24.1551) (-23.0053, 24.1655) (-23.0174, 24.1655) knots 0 0 0 1 1 1
  spline S254 degree 2 poles (-23.0174, 24.1655) (-23.0278, 24.1655) (-23.0875, 24.1491) (-23.0935, 24.1439) knots 0 0 0 1 2 2 2
  spline S255 degree 2 poles (-23.0935, 24.1439) (-23.4249, 23.829) (-23.5399, 23.829) knots 0 0 0 1 1 1
  spline S256 degree 2 poles (-23.5399, 23.829) (-23.5486, 23.829) (-23.5486, 23.8385) knots 0 0 0 1 1 1
  spline S257 degree 2 poles (-23.5486, 23.8385) (-23.5486, 23.8515) (-23.5295, 23.8549) knots 0 0 0 1 1 1
  spline S258 degree 2 poles (-23.5295, 23.8549) (-23.5062, 23.8593) (-23.4672, 23.8774) knots 0 0 0 1 1 1
  spline S259 degree 2 poles (-23.4672, 23.8774) (-23.4093, 23.9025) (-23.2951, 23.9985) knots 0 0 0 1 1 1
  spline S260 degree 2 poles (-23.2951, 23.9985) (-23.193, 24.0833) (-23.1377, 24.1447) knots 0 0 0 1 1 1
  line L56 (-22.6558, 24.1482) -> (-22.8833, 23.9596)
  spline S261 degree 2 poles (-22.8833, 23.9596) (-23.0555, 23.829) (-23.1247, 23.829) knots 0 0 0 1 1 1
  spline S262 degree 2 poles (-23.1247, 23.829) (-23.1333, 23.829) (-23.1333, 23.8385) knots 0 0 0 1 1 1
  spline S263 degree 2 poles (-23.1333, 23.8385) (-23.1333, 23.8515) (-23.1186, 23.8549) knots 0 0 0 1 1 1
  spline S264 degree 2 poles (-23.1186, 23.8549) (-23.0667, 23.8679) (-23.0382, 23.8835) knots 0 0 0 1 1 1
  spline S265 degree 2 poles (-23.0382, 23.8835) (-22.9932, 23.9068) (-22.8496, 24.021) knots 0 0 0 1 1 1
  spline S266 degree 2 poles (-22.8496, 24.021) (-22.7847, 24.0712) (-22.6627, 24.1819) knots 0 0 0 1 1 1
  spline S267 degree 2 poles (-22.6627, 24.1819) (-22.6169, 24.2295) (-22.597, 24.2295) knots 0 0 0 1 1 1
  spline S268 degree 2 poles (-22.597, 24.2295) (-22.5572, 24.2295) (-22.5572, 24.2036) knots 0 0 0 1 1 1
  spline S269 degree 2 poles (-22.5572, 24.2036) (-22.5572, 24.1707) (-22.6377, 24.0677) knots 0 0 0 1 1 1
  spline S270 degree 2 poles (-22.6377, 24.0677) (-22.482, 24.2105) (-22.4231, 24.2105) knots 0 0 0 1 1 1
  spline S271 degree 2 poles (-22.4231, 24.2105) (-22.4032, 24.2105) (-22.3704, 24.1854) (-22.3704, 24.1664) knots 0 0 0 1 2 2 2
  spline S272 degree 2 poles (-22.3704, 24.1664) (-22.3704, 24.1378) (-22.4093, 24.0825) knots 0 0 0 1 1 1
  spline S273 degree 2 poles (-22.4093, 24.0825) (-22.2648, 24.2252) (-22.1818, 24.2252) knots 0 0 0 1 1 1
  spline S274 degree 2 poles (-22.1818, 24.2252) (-22.1342, 24.2252) (-22.1342, 24.1863) knots 0 0 0 1 1 1
  spline S275 degree 2 poles (-22.1342, 24.1863) (-22.1342, 24.1361) (-22.3686, 23.8956) (-22.3686, 23.8714) knots 0 0 0 1 2 2 2
  spline S276 degree 2 poles (-22.3686, 23.8714) (-22.3686, 23.8532) (-22.3185, 23.8523) (-22.3185, 23.8411) knots 0 0 0 1 2 2 2
  spline S277 degree 2 poles (-22.3185, 23.8411) (-22.3185, 23.8273) (-22.36, 23.8273) knots 0 0 0 1 1 1
  spline S278 degree 2 poles (-22.36, 23.8273) (-22.4162, 23.8273) (-22.4162, 23.8766) knots 0 0 0 1 1 1
  spline S279 degree 2 poles (-22.4162, 23.8766) (-22.4162, 23.9319) (-22.2121, 24.1638) (-22.2121, 24.1776) knots 0 0 0 1 2 2 2
  spline S280 degree 2 poles (-22.2121, 24.1776) (-22.2121, 24.1863) (-22.2224, 24.1863) knots 0 0 0 1 1 1
  spline S281 degree 2 poles (-22.2224, 24.1863) (-22.2657, 24.1863) (-22.4093, 24.0513) knots 0 0 0 1 1 1
  spline S282 degree 2 poles (-22.4093, 24.0513) (-22.5287, 23.9397) (-22.5849, 23.8705) knots 0 0 0 1 1 1
  spline S283 degree 2 poles (-22.5849, 23.8705) (-22.6195, 23.8273) (-22.6359, 23.8273) knots 0 0 0 1 1 1
  spline S284 degree 2 poles (-22.6359, 23.8273) (-22.6636, 23.8273) (-22.6636, 23.8532) knots 0 0 0 1 1 1
  spline S285 degree 2 poles (-22.6636, 23.8532) (-22.6636, 23.8792) (-22.4396, 24.1292) (-22.4396, 24.1586) knots 0 0 0 1 2 2 2
  spline S286 degree 2 poles (-22.4396, 24.1586) (-22.4396, 24.1716) (-22.4534, 24.1716) knots 0 0 0 1 1 1
  spline S287 degree 2 poles (-22.4534, 24.1716) (-22.4906, 24.1716) (-22.623, 24.047) knots 0 0 0 1 1 1
  spline S288 degree 2 poles (-22.623, 24.047) (-22.7363, 23.9406) (-22.783, 23.88) knots 0 0 0 1 1 1
  spline S289 degree 2 poles (-22.783, 23.88) (-22.8193, 23.8333) (-22.8461, 23.8333) knots 0 0 0 1 1 1
  spline S290 degree 2 poles (-22.8461, 23.8333) (-22.8704, 23.8333) (-22.8704, 23.8549) knots 0 0 0 1 1 1
  spline S291 degree 2 poles (-22.8704, 23.8549) (-22.8704, 23.8818) (-22.7709, 24.0055) knots 0 0 0 1 1 1
  line L57 (-22.7709, 24.0055) -> (-22.6558, 24.1482)
  spline S292 degree 2 poles (-22.0667, 23.9795) (-22.2579, 23.829) (-22.3297, 23.829) knots 0 0 0 1 1 1
  spline S293 degree 2 poles (-22.3297, 23.829) (-22.3384, 23.829) (-22.3384, 23.8385) knots 0 0 0 1 1 1
  spline S294 degree 2 poles (-22.3384, 23.8385) (-22.3384, 23.8523) (-22.3211, 23.8549) knots 0 0 0 1 1 1
  spline S295 degree 2 poles (-22.3211, 23.8549) (-22.2544, 23.8653) (-22.1351, 23.9587) knots 0 0 0 1 1 1
  line L58 (-22.1351, 23.9587) -> (-22.0434, 24.0305)
  line L59 (-22.0434, 24.0305) -> (-21.8954, 24.1482)
  spline S296 degree 2 poles (-21.8954, 24.1482) (-21.7942, 24.2183) (-21.7216, 24.2183) knots 0 0 0 1 1 1
  spline S297 degree 2 poles (-21.7216, 24.2183) (-21.6679, 24.2183) (-21.6619, 24.1646) knots 0 0 0 1 1 1
  spline S298 degree 2 poles (-21.6619, 24.1646) (-21.6342, 24.1914) (-21.623, 24.1914) knots 0 0 0 1 1 1
  spline S299 degree 2 poles (-21.623, 24.1914) (-21.5996, 24.1914) (-21.5996, 24.1716) knots 0 0 0 1 1 1
  spline S300 degree 2 poles (-21.5996, 24.1716) (-21.5996, 24.1465) (-21.8185, 23.8913) (-21.8185, 23.8696) knots 0 0 0 1 2 2 2
  spline S301 degree 2 poles (-21.8185, 23.8696) (-21.8185, 23.8549) (-21.7726, 23.8532) (-21.7726, 23.842) knots 0 0 0 1 2 2 2
  spline S302 degree 2 poles (-21.7726, 23.842) (-21.7726, 23.8273) (-21.8202, 23.8273) knots 0 0 0 1 1 1
  spline S303 degree 2 poles (-21.8202, 23.8273) (-21.8678, 23.8273) (-21.8678, 23.8696) knots 0 0 0 1 1 1
  spline S304 degree 2 poles (-21.8678, 23.8696) (-21.8678, 23.9034) (-21.8297, 23.9648) knots 0 0 0 1 1 1
  line L60 (-21.8297, 23.9648) -> (-21.9179, 23.8895)
  spline S305 degree 2 poles (-21.9179, 23.8895) (-21.9828, 23.8411) (-22.0217, 23.8411) knots 0 0 0 1 1 1
  spline S306 degree 2 poles (-22.0217, 23.8411) (-22.0832, 23.8411) (-22.0832, 23.9034) knots 0 0 0 1 1 1
  spline S307 degree 2 poles (-22.0832, 23.9034) (-22.0832, 23.938) (-22.0667, 23.9795) knots 0 0 0 1 1 1
  spline S308 degree 2 poles (-21.7121, 24.1889) (-21.7544, 24.1889) (-22.0183, 23.9371) (-22.0183, 23.8947) knots 0 0 0 1 2 2 2
  spline S309 degree 2 poles (-22.0183, 23.8947) (-22.0183, 23.8757) (-22.0001, 23.8757) knots 0 0 0 1 1 1
  spline S310 degree 2 poles (-22.0001, 23.8757) (-21.9586, 23.8757) (-21.6913, 24.1222) (-21.6913, 24.1655) knots 0 0 0 1 2 2 2
  spline S311 degree 2 poles (-21.6913, 24.1655) (-21.6913, 24.1889) (-21.7121, 24.1889) knots 0 0 0 1 1 1
  spline S312 degree 2 poles (-21.3081, 24.0453) (-21.1117, 24.2113) (-21.033, 24.2113) knots 0 0 0 1 1 1
  spline S313 degree 2 poles (-21.033, 24.2113) (-20.982, 24.2113) (-20.982, 24.1638) knots 0 0 0 1 1 1
  spline S314 degree 2 poles (-20.982, 24.1638) (-20.982, 24.1214) (-21.2112, 23.9008) (-21.2112, 23.8783) knots 0 0 0 1 2 2 2
  spline S315 degree 2 poles (-21.2112, 23.8783) (-21.2112, 23.8549) (-21.1593, 23.8515) (-21.1593, 23.8411) knots 0 0 0 1 2 2 2
  spline S316 degree 2 poles (-21.1593, 23.8411) (-21.1593, 23.8273) (-21.2112, 23.8273) knots 0 0 0 1 1 1
  spline S317 degree 2 poles (-21.2112, 23.8273) (-21.2709, 23.8273) (-21.2709, 23.88) knots 0 0 0 1 1 1
  spline S318 degree 2 poles (-21.2709, 23.88) (-21.2709, 23.9241) (-21.2138, 23.9925) knots 0 0 0 1 1 1
  spline S319 degree 2 poles (-21.2138, 23.9925) (-21.1844, 24.0271) (-21.1082, 24.0998) knots 0 0 0 1 1 1
  spline S320 degree 2 poles (-21.1082, 24.0998) (-21.0512, 24.1543) (-21.0512, 24.1655) knots 0 0 0 1 1 1
  spline S321 degree 2 poles (-21.0512, 24.1655) (-21.0512, 24.175) (-21.0641, 24.175) knots 0 0 0 1 1 1
  spline S322 degree 2 poles (-21.0641, 24.175) (-21.1048, 24.175) (-21.2406, 24.066) knots 0 0 0 1 1 1
  spline S323 degree 2 poles (-21.2406, 24.066) (-21.3548, 23.9761) (-21.4093, 23.9181) knots 0 0 0 1 1 1
  spline S324 degree 2 poles (-21.4093, 23.9181) (-21.4794, 23.8446) (-21.4941, 23.8446) knots 0 0 0 1 1 1
  spline S325 degree 2 poles (-21.4941, 23.8446) (-21.5062, 23.8446) (-21.5243, 23.8671) (-21.5243, 23.8792) knots 0 0 0 1 2 2 2
  spline S326 degree 2 poles (-21.5243, 23.8792) (-21.5243, 23.8956) (-21.4257, 24.0115) knots 0 0 0 1 1 1
  line L61 (-21.4257, 24.0115) -> (-21.3081, 24.1499)
  line L62 (-21.3081, 24.1499) -> (-21.4906, 24.002)
  line L63 (-21.4906, 24.002) -> (-21.6255, 23.8991)
  spline S327 degree 2 poles (-21.6255, 23.8991) (-21.7285, 23.829) (-21.783, 23.829) knots 0 0 0 1 1 1
  spline S328 degree 2 poles (-21.783, 23.829) (-21.7925, 23.829) (-21.7925, 23.8376) knots 0 0 0 1 1 1
  spline S329 degree 2 poles (-21.7925, 23.8376) (-21.7925, 23.8506) (-21.7726, 23.8549) knots 0 0 0 1 1 1
  spline S330 degree 2 poles (-21.7726, 23.8549) (-21.7458, 23.8601) (-21.7086, 23.8766) knots 0 0 0 1 1 1
  spline S331 degree 2 poles (-21.7086, 23.8766) (-21.6567, 23.8991) (-21.4967, 24.0288) knots 0 0 0 1 1 1
  spline S332 degree 2 poles (-21.4967, 24.0288) (-21.3522, 24.1456) (-21.289, 24.207) knots 0 0 0 1 1 1
  spline S333 degree 2 poles (-21.289, 24.207) (-21.2778, 24.2183) (-21.2553, 24.233) knots 0 0 0 1 1 1
  spline S334 degree 2 poles (-21.2553, 24.233) (-21.2441, 24.2373) (-21.2311, 24.2373) knots 0 0 0 1 1 1
  spline S335 degree 2 poles (-21.2311, 24.2373) (-21.219, 24.2373) (-21.1939, 24.2209) (-21.1939, 24.2096) knots 0 0 0 1 2 2 2
  spline S336 degree 2 poles (-21.1939, 24.2096) (-21.1939, 24.1966) (-21.3081, 24.0453) knots 0 0 0 1 1 1
  point P0 (0, 0)
  constraints: 2 other
emboss "Emboss1" sketch "Sketch2" operation cut depth 1 direction (0, 0, -1)
body "Solid1"
